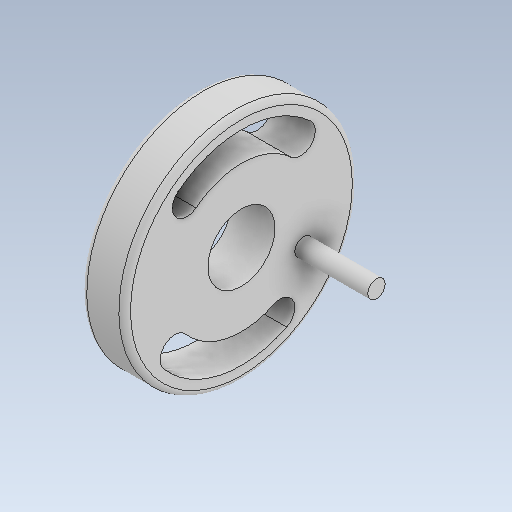
# Autodesk Inventor part: compression wheel
Saved by Autodesk Inventor 2021 (Build 250183000, 183)
## iProperties
Created: 2021-07-03
Part Number: compression wheel
Material: Generic
Document SubType Name: Modeling
Designer: Dell
Density: 1 g/cm^3
Appearance: Default
Author: Dell
Autodesk Inventor part; units mm, degrees
ref_plane "YZ Plane" through (0, 0, 0) normal (1, 0, 0) x (0, 1, 0)
ref_plane "XZ Plane" through (0, 0, 0) normal (0, 1, 0) x (-1, 0, 0)
ref_plane "XY Plane" through (0, 0, 0) normal (0, 0, 1) x (1, 0, 0)
sketch "Sketch1" plane through (0, 0, 0) normal (1, 0, 0) x (0, 1, 0)
  circle A0 centre (0, 0) radius 4
  dimension "d0" = 8
  constraints: 1 centre point, 1 coincident
  measures "d0" diameter of A0
extrude "Extrusion1" add sketch "Sketch1" along normal blind 1.5
sketch "Sketch2" plane through (1.5, 0, 0) normal (1, 0, 0) x (0, 0, -1)
  circle A0 centre (0, 0) radius 1.15
  arc A1 (-2.1791, 2.7389) -> (-1.5565, 1.9564) centre (-1.8678, 2.3476) ccw
  arc A2 (1.6939, 1.8387) -> (2.3714, 2.5742) centre (2.0326, 2.2065) ccw
  arc A3 (-1.9044, -1.6196) -> (-2.6662, -2.2675) centre (-2.2853, -1.9435) ccw
  arc A4 (1.5526, -3.1368) -> (1.109, -2.2406) centre (1.3308, -2.6887) ccw
  arc A5 (-1.9044, -1.6196) -> (1.109, -2.2406) centre (0, 0) ccw
  arc A6 (1.6939, 1.8387) -> (-1.5565, 1.9564) centre (0, 0) ccw
  arc A7 (-2.6662, -2.2675) -> (1.5526, -3.1368) centre (0, 0) ccw
  arc A8 (2.3714, 2.5742) -> (-2.1791, 2.7389) centre (0, 0) ccw
  dimension "d5" = 2.3
  dimension "d6" = 1
  dimension "d7" = 1
  dimension "d8" = 1
  dimension "d9" = 1
  constraints: 16 point on circle, 9 centre point, 3 coincident
  measures "d5" diameter of A0
  measures "d6" diameter of A1
  measures "d7" diameter of A2
  measures "d8" diameter of A3
  measures "d9" diameter of A4
extrude "Extrusion2" cut sketch "Sketch2" against normal blind 2
fillet "Fillet1" radius 0.2 1 edges at (1.5, -4, 0)
fillet "Fillet2" radius 0.2 1 edges at (0, -4, 0)
sketch "Sketch6" plane through (1.5, 0, 0) normal (1, 0, 0) x (0, 0, -1)
  circle A0 centre (2.1297, -1.0387) radius 0.3
  point P0 (0, 0)
  dimension "d20" = 0.6
  constraints: 1 centre point
  measures "d20" diameter of A0
extrude "Extrusion5" add sketch "Sketch6" along normal blind 2.5
sketch "Sketch7" plane through (0, 0, 0) normal (-1, 0, 0) x (0, 0, 1)
  point P0 (0, 0)
body "Solid1"
